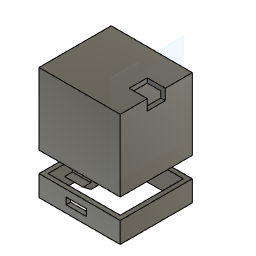
Cover_BoxAndBase (Autodesk Fusion 360 design; units mm, degrees)
Autodesk Fusion 360 part; units mm, degrees
sketch "Sketch1" plane through (0, 0, 0) normal (1, 0, 0) x (0, 1, 0)
  line L0 (0, 0) -> (14.12, 0)
  line L1 (14.12, 0) -> (14.12, 18.38)
  line L2 (14.12, 18.38) -> (0, 18.38)
  line L3 (0, 18.38) -> (0, 0)
  dimension "d1" = 14.12
  dimension "d2" = 18.38
  constraint horizontal L0
  constraint vertical L1
  constraint horizontal L2
  constraint vertical L3
  constraint coincident L0.start L3.end
  measures "d1" distance of L0.start L0.end
  measures "d2" distance of L0.start L2.end
sketch "Sketch2" plane through (6, 0, 0) normal (1, 0, 0) x (0, 1, 0)
  line L0 (0, 18.38) -> (0, 0)
  line L1 (0, 0) -> (14.12, 0)
  line L2 (14.12, 0) -> (14.12, 18.38)
  line L3 (14.12, 18.38) -> (0, 18.38)
  line L4 (2, 2) -> (12.12, 2)
  line L5 (12.12, 2) -> (12.12, 16.38)
  line L6 (12.12, 16.38) -> (2, 16.38)
  line L7 (2, 16.38) -> (2, 2)
  dimension "d5" = -2
sketch "Sketch3" plane through (6, 0, 0) normal (1, 0, 0) x (0, 1, 0)
  line L0 (12.12, 2) -> (2, 2)
  line L1 (2, 2) -> (2, 16.38)
  line L2 (2, 16.38) -> (12.12, 16.38)
  line L3 (12.12, 16.38) -> (12.12, 2)
  line L4 (0, 18.38) -> (0, 0)
  line L5 (0, 0) -> (14.12, 0)
  line L6 (14.12, 0) -> (14.12, 18.38)
  line L7 (14.12, 18.38) -> (0, 18.38)
  line L8 (8.435, 16.4238) -> (5.685, 16.4238)
  line L9 (5.685, 16.4238) -> (5.685, 18.4238)
  line L10 (5.685, 18.4238) -> (8.435, 18.4238)
  line L11 (8.435, 18.4238) -> (8.435, 16.4238)
  line L12 (8.435, 16.4238) -> (5.685, 18.4238) construction
  line L13 (5.685, 16.4238) -> (8.435, 18.4238) construction
  point P0 (7.06, 17.4238)
  dimension "d8" = 2.75
  dimension "d9" = 2
  constraint horizontal L8
  constraint perpendicular L8 L9
  constraint parallel L8 L10
  constraint parallel L9 L11
  constraint coincident L12 P0
  constraint coincident L13 P0
  measures "d8" distance of L9.end L10.end
  measures "d9" distance of L8.end L9.end
sketch "Sketch4" plane through (0, 0, 0) normal (0, -1, 0) x (1, 0, 0)
  line L0 (0, 18.38) -> (0, 0)
  line L1 (0, 0) -> (6, 0)
  line L2 (6, 0) -> (6, 18.38)
  line L3 (6, 18.38) -> (0, 18.38)
  line L4 (1238, -32) -> (1239, -32)
  line L5 (1239, -32) -> (1239, -46.38)
  line L6 (1239, -46.38) -> (1238, -46.38)
  line L7 (1238, -46.38) -> (1238, -32)
  line L8 (-15, 12.38) -> (-16, 12.38)
  line L9 (-16, 12.38) -> (-16, -2)
  line L10 (-16, -2) -> (-15, -2)
  line L11 (-15, -2) -> (-15, 12.38)
  dimension "d14" = 1
  dimension "d15" = 14.38
  dimension "d16" = 1
  dimension "d17" = 14.38
  constraint horizontal L4
  constraint vertical L5
  constraint horizontal L6
  constraint vertical L7
  constraint vertical L9
  constraint perpendicular L8 L9
  constraint horizontal L10
  constraint parallel L9 L11
  measures "d14" distance of L4.start L4.end
  measures "d15" distance of L4.start L6.end
  measures "d16" distance of L8.start L8.end
  measures "d17" distance of L8.start L10.end
sketch "Sketch5" plane through (0, 0, 2) normal (0, 0, 1) x (-1, 0, 0)
  line L0 (-6, -2) -> (-6, -12.12)
  line L1 (-6, -12.12) -> (0, -12.12)
  line L2 (0, -2) -> (-6, -2)
  line L3 (0, -12.12) -> (0, -2)
sketch "Sketch6" plane through (4, 0, 0) normal (1, 0, 0) x (0, 1, 0)
  line L0 (5.685, 18.38) -> (5.685, 16.38)
  line L1 (5.685, 16.38) -> (8.435, 16.38)
  line L2 (8.435, 16.38) -> (8.435, 18.38)
  line L3 (8.435, 18.38) -> (5.685, 18.38)
  line L4 (12.1332, 16.38) -> (12.1332, 1.9861)
  line L5 (12.1336, 16.4249, -4) -> (2.0136, 16.4249, -4)
  line L6 (2.0136, 16.4249, -4) -> (2.0136, 18.4249, -4)
  line L7 (2.0136, 18.4249, -4) -> (12.1336, 18.4249, -4)
  line L8 (12.1336, 18.4249, -4) -> (12.1336, 16.4249, -4)
  dimension "d20" = 10.12
  dimension "d21" = 2
  constraint vertical L4
sketch "Sketch7" plane through (0, 2, 0) normal (0, 1, 0) x (-1, 0, 0)
  line L0 (0, 16.38) -> (-6, 16.38)
  line L1 (-6, 16.38) -> (-6, 2)
  line L2 (-6, 2) -> (0, 2)
  line L3 (0, 2) -> (0, 16.38)
  line L4 (0, 13) -> (-1, 13)
  line L5 (-1, 13) -> (-1, 11)
  line L6 (-1, 11) -> (0, 11)
  line L7 (0, 11) -> (0, 13)
  constraint horizontal L4
  constraint vertical L5
  constraint horizontal L6
  constraint vertical L7
  constraint coincident L3 L4.start
sketch "Sketch8" plane through (0, 2, 0) normal (0, 1, 0) x (-1, 0, 0)
  line L0 (-1, 13) -> (0, 13)
  line L1 (0, 13) -> (0, 16.38)
  line L2 (0, 16.38) -> (-6, 16.38)
  line L3 (-6, 16.38) -> (-6, 2)
  line L4 (-6, 2) -> (0, 2)
  line L5 (0, 2) -> (0, 11)
  line L6 (0, 11) -> (-1, 11)
  line L7 (-1, 11) -> (-1, 13)
  line L8 (-1, 13) -> (-2, 13)
  line L9 (-2, 13) -> (-2, 15.5114)
  line L10 (-2, 15.5114) -> (-1, 15.5114)
  line L11 (-1, 15.5114) -> (-1, 13)
  dimension "d26" = 1
  constraint horizontal L8
  constraint vertical L9
  constraint horizontal L10
  constraint vertical L11
  constraint coincident L0.start L7.end
  measures "d26" distance of L0.start L8.end
sketch "Sketch9" plane through (0, 8.435, 0) normal (0, -1, 0) x (1, 0, 0)
  line L0 (4, 18.38) -> (4, 16.38)
  line L1 (4, 16.38) -> (6, 16.38)
  line L2 (6, 16.38) -> (6, 18.38)
  line L3 (6, 18.38) -> (4, 18.38)
  line L4 (4.1228, 1.37) -> (4.6228, 1.37)
  line L5 (4.6228, 1.37) -> (4.6228, 16.37)
  line L6 (4.6228, 16.37) -> (4.1228, 16.37)
  line L7 (4.1228, 16.37) -> (4.1228, 1.37)
  dimension "d33" = 0.5
  dimension "d34" = 15
  constraint horizontal L4
  constraint vertical L5
  constraint horizontal L6
  constraint vertical L7
  measures "d33" distance of L4.start L4.end
  measures "d34" distance of L4.start L6.end
sketch "Sketch10" plane through (0, 0, 16.38) normal (0, 0, -1) x (1, 0, 0)
  line L0 (2, -2.0136) -> (2, -12.12)
  line L1 (2, -12.12) -> (6, -12.12)
  line L2 (6, -12.12) -> (6, -8.435)
  line L3 (6, -8.435) -> (4, -8.435)
  line L4 (4, -8.435) -> (4, -5.685)
  line L5 (4, -5.685) -> (6, -5.685)
  line L6 (6, -5.685) -> (6, -2)
  line L7 (6, -2) -> (0, -2)
  line L8 (0, -2) -> (0, -2.0136)
  line L9 (0, -2.0136) -> (2, -2.0136)
  line L10 (-1, 5) -> (12, 5)
  line L11 (12, 5) -> (12, 21)
  line L12 (12, 21) -> (-1, 21)
  line L13 (-1, 21) -> (-1, 5)
  dimension "d39" = 13
  constraint horizontal L10
  constraint vertical L11
  constraint horizontal L12
  constraint vertical L13
  measures "d39" distance of L10.start L10.end
extrude "Extrude11" add sketch "Sketch10" along normal blind 20.5 contours L10 L11 L12 L13 makes body 1
sketch "Sketch11" plane through (0, 0, -4.12) normal (0, 0, -1) x (1, 0, 0)
  line L0 (-1, 21) -> (-1, 5)
  line L1 (-1, 5) -> (12, 5)
  line L2 (12, 5) -> (12, 21)
  line L3 (12, 21) -> (-1, 21)
  line L4 (0, 6) -> (11, 6)
  line L5 (11, 6) -> (11, 20)
  line L6 (11, 20) -> (0, 20)
  line L7 (0, 20) -> (0, 6)
  constraint horizontal L4
  constraint vertical L5
  constraint horizontal L6
  constraint vertical L7
extrude "Extrude12" cut sketch "Sketch11" against normal blind 19.5 contours L4 L5 L6 L7 bodies 1
sketch "Sketch12" plane through (0, 0, 0) normal (0, 0, 1) x (1, 0, 0)
  line L0 (12.1825, -11, 14) -> (8, -11, 14)
  line L1 (8, -11, 14) -> (8, -15, 14)
  line L2 (8, -15, 14) -> (12.1825, -15, 14)
  line L3 (12.1825, -15, 14) -> (12.1825, -11, 14)
extrude "Extrude13" cut sketch "Sketch12" along normal blind 5 contours L0 L1 L2 L3 in plane through (0, 0, 14) normal (0, 0, 1) bodies 1
sketch "Sketch13" plane through (0, 0, 16.38) normal (0, 0, 1) x (-1, 0, 0)
  line L0 (-12, 15) -> (-8, 15)
  line L1 (-8, 15) -> (-8, 11)
  line L2 (-8, 11) -> (-12, 11)
  line L3 (-12, 11) -> (-12, 5)
  line L4 (-12, 5) -> (1, 5)
  line L5 (1, 5) -> (1, 21)
  line L6 (1, 21) -> (-12, 21)
  line L7 (-12, 21) -> (-12, 15)
  line L8 (1, 6) -> (-4.6, 6)
  line L9 (-4.6, 6) -> (-4.6, 20)
  line L10 (-4.6, 20) -> (1, 20)
  line L11 (1, 20) -> (1, 6)
  dimension "d46" = 5.6
  dimension "d47" = 14
  constraint horizontal L8
  constraint vertical L9
  constraint horizontal L10
  constraint vertical L11
  measures "d46" distance of L8.start L8.end
  measures "d47" distance of L8.start L10.end
extrude "Extrude14" add sketch "Sketch13" along normal blind 11 contours L5 L8 L9 L10 L11 bodies 1
extrude "Extrude15" cut 1 faces at (2.7333, -15.3333, 27.38) along direction (0, 0, -1) blind 22 on bodies 1 bodies 1
extrude "Extrude16" add 1 faces at (12, -13.6667, 1.92) along direction (1, 0, 0) blind 5 on bodies 1 bodies 1
extrude "Extrude17" cut 1 faces at (11, -12.3333, 1.92) along direction (1, 0, 0) blind 5 on bodies 1 bodies 1
extrude "Extrude18" add 1 faces at (8, -12.3333, 16.0467) along direction (1, 0, 0) blind 5 on bodies 1 bodies 1
extrude "Extrude19" add 1 faces at (4.6, -15.3333, 15.7133) along direction (-1, 0, 0) blind 4 on bodies 1 bodies 1
extrude "Extrude20" add 1 faces at (0.6, -15.3333, 15.7133) along direction (-1, 0, 0) blind 1.6 on bodies 1 bodies 1
extrude "Extrude21" add 1 faces at (-0.3333, -15.3333, 5.38) along direction (0, 0, 1) blind 10 on bodies 1 bodies 1
box "BoxPrimitive1" add length 14 width 1 height 0.5 placed x (0, 1, 0) y (-1, 0, 0) z (0, 0, 1) at (9.5, -20, 0) bodies 1
extrude "Extrude23" add 1 faces at (8.8333, -15.3333, 0.5) along direction (0, 0, 1) blind 15.5 on bodies 1 bodies 1
extrude "Extrude24" cut 1 faces at (8.8333, -15.3333, 0) along direction (0, 0, 1) blind 7.5 on bodies 1 bodies 1
extrude "Extrude25" add 1 faces at (8.8333, -15.3333, 7.5) along direction (0, 0, -1) blind 2.5 on bodies 1 bodies 1
sketch "Sketch15" plane through (0, 0, 0) normal (1, 0, 0) x (0, 1, 0)
sketch "Sketch16" plane through (17, 0, 0) normal (1, 0, 0) x (0, 1, 0)
  line L0 (-15, 14) -> (-15, 16.38)
  line L1 (-15, 16.38) -> (-21, 16.38)
  line L2 (-21, 16.38) -> (-21, -4.12)
  line L3 (-21, -4.12) -> (-5, -4.12)
  line L4 (-5, -4.12) -> (-5, 16.38)
  line L5 (-5, 16.38) -> (-11, 16.38)
  line L6 (-11, 16.38) -> (-11, 14)
  line L7 (-11, 14) -> (-15, 14)
box "BoxPrimitive2" add length 0.5 width 18 height 0.5 placed x (0, 0, 1) y (-1, 0, 0) z (0, -1, 0) at (17, -21, 0) bodies 1
extrude "Extrude26" cut 1 faces at (5, -21.5, 0.1667) along direction (0, 1, 0) blind 16.5 on bodies 1 bodies 1 makes body 2 at (11, -5, 5.7933)
extrude "Extrude27" add 1 faces at (10.6667, -5.3333, -4.12) along direction (0, 0, -1) blind 0.5 on bodies 1 bodies 1
box "BoxPrimitive3" add length 1.5 width 3 height 1 placed x (0, 0, 1) y (-1, 0, 0) z (0, -1, 0) at (8, -21, -3) bodies 1
extrude "Extrude28" cut 1 faces at (6, -22, -2.5) along direction (0, 1, 0) blind 20 on bodies 1 bodies 1
box "BoxPrimitive4" add length 1.5 width 3 height 2 placed x (0, 0, 1) y (-1, 0, 0) z (0, -1, 0) at (7.9158, -6, 0.5) bodies 2
extrude "Extrude29" cut 1 faces at (4.9158, -6.6667, 1.5) along direction (1, 0, 0) blind 0.2 on bodies 2 bodies 2
extrude "Extrude30" cut 1 faces at (7.9158, -6.6667, 1.5) along direction (-1, 0, 0) blind 0.2 on bodies 2 bodies 2
box "BoxPrimitive5" add length 0.2 width 2.6 height 1 placed x (0, -1, 0) y (-1, 0, 0) z (0, 0, -1) at (7.7158, -6, 0.5) bodies 1 2
extrude "Extrude31" cut 1 faces at (5.9824, -6.0667, -0.5) along direction (0, 0, 1) blind 1.2 on bodies 1 bodies 1 makes body 3 at (11, -5, 5.7933)
extrude "Extrude32" add 1 faces at (6.8491, -7.4, 0.5) along direction (0, 0, -1) blind 2.4 on bodies 3 bodies 3
extrude "Extrude33" add 1 faces at (6.8491, -7.4, -1.9) along direction (0, 0, -1) blind 0.5 on bodies 3 bodies 3
box "BoxPrimitive6" add length 1.5 width 3 height 2 placed x (0, 0, 1) y (1, 0, 0) z (0, 1, 0) at (5, -20, 0.5) bodies 3
extrude "Extrude34" cut 1 faces at (8, -19.3333, 1.5) along direction (-1, 0, 0) blind 0.2 on bodies 3 bodies 3
extrude "Extrude35" cut 1 faces at (5, -19.3333, 1.5) along direction (1, 0, 0) blind 0.2 on bodies 3 bodies 3
box "BoxPrimitive7" add length 0.2 width 2.6 height 0.2 placed x (0, 1, 0) y (1, 0, 0) z (0, 0, -1) at (5.2, -20, 0.5) bodies 3
extrude "Extrude36" cut 1 faces at (6.9333, -19.9333, 0.3) along direction (0, 0, 1) blind 0.4 on bodies 3 bodies 3
extrude "Extrude37" add 1 faces at (6.0667, -19.2, 0.5) along direction (0, 0, -1) blind 3.1 on bodies 3 bodies 3
extrude "Extrude38" cut 1 faces at (6.0667, -19.2, -2.6) along direction (0, 0, 1) blind 0.1 on bodies 3 bodies 3
move_body "Move2" bodies 1 to x (1, 0, 0) y (0, 1, 0) z (0, 0, 1) at (0, 0, -3)
move_body "Move3" bodies 3 to x (1, 0, 0) y (0, 1, 0) z (0, 0, 1) at (0, -6, 0)
move_body "Move4" bodies 1 to x (1, 0, 0) y (0, 1, 0) z (0, 0, 1) at (0, -6, 0)
move_body "Move5" bodies 1 to x (1, 0, 0) y (0, 1, 0) z (0, 0, 1) at (8, 0, 0)
move_body "Move6" bodies 3 to x (1, 0, 0) y (0, 1, 0) z (0, 0, 1) at (8, 0, 0)
move_body "Move7" bodies 1 to x (1, 0, 0) y (0, 1, 0) z (0, 0, 1) at (-13, 0, 0)
sketch "Sketch23" plane through (15.8, 0, 0) normal (1, 0, 0) x (0, 1, 0)
  line L0 (-25.8, -2.5) -> (-24, -2.5)
  line L1 (-24, -2.5) -> (-24, 2)
  line L2 (-24, 2) -> (-26, 2)
  line L3 (-26, 2) -> (-26, 0.7)
  line L4 (-26, 0.7) -> (-25.8, 0.7)
  line L5 (-25.8, 0.7) -> (-25.8, -2.5)
  line L6 (-27.8, -1) -> (-25.8, -1)
  line L7 (-25.8, -1) -> (-25.8, -2.5)
  line L8 (-27.8, -1) -> (-25.8, -2.5)
  dimension "d134" = 1.5
  constraint horizontal L6
  constraint vertical L7
  constraint coincident L0.start L5.end
  measures "d134" distance of L0.start L6.end
extrude "Extrude39" add sketch "Sketch23" against normal blind 2.6 contours L5 L6 L7 L8 bodies 3
sketch "Sketch24" plane through (13.1158, 0, 0) normal (-1, 0, 0) x (0, -1, 0)
  line L0 (12.2, 0.7) -> (12.2, -2.4)
  line L1 (12.2, -2.4) -> (14, -2.4)
  line L2 (14, -2.4) -> (14, 2)
  line L3 (14, 2) -> (12, 2)
  line L4 (12, 2) -> (12, 0.7)
  line L5 (12, 0.7) -> (12.2, 0.7)
  line L6 (10.2, -0.9) -> (12.2, -0.9)
  line L7 (12.2, -0.9) -> (12.2, -2.4)
  line L8 (10.2, -0.9) -> (12.2, -2.4)
  dimension "d138" = 1.5
  constraint horizontal L6
  constraint vertical L7
  constraint coincident L0.end L1.start
  measures "d138" distance of L0.end L6.end
extrude "Extrude40" add sketch "Sketch24" against normal blind 2.6 contours L0 L6 L7 L8 bodies 3
extrude "Extrude41" cut 1 faces at (13.9824, -10.8667, -0.9) along direction (0, 0, -1) blind 0.2 on bodies 3 bodies 3
extrude "Extrude42" cut 1 faces at (14.9333, -27.1333, -1) along direction (0, 0, -1) blind 0.2 on bodies 3 bodies 3
move_body "Move8" bodies 1 to x (1, 0, 0) y (0, 1, 0) z (0, 0, 1) at (13, 0, -1)
copy_body "Body->Comp1" bodies 3 removing the originals makes body 4 in component "Component"
extrude "Extrude1" add 1 faces at (17.5, -16.6667, 9.2933) along direction (1, 0, 0) blind 1.5 on bodies 4 bodies 4 in component "Component"
extrude "Extrude2" cut 1 faces at (16.5, -16.6667, 9.2933) along direction (1, 0, 0) blind 1.5 on bodies 4 bodies 4 in component "Component"
extrude "Extrude3" add 1 faces at (15.8, -24.6, 0.0667) along direction (1, 0, 0) blind 1.5 on bodies 4 bodies 4 in component "Component"
extrude "Extrude4" add 1 faces at (15.7158, -13.4, -0.5) along direction (1, 0, 0) blind 1.5 on bodies 4 bodies 4 in component "Component"
extrude "Extrude43" cut 1 faces at (16, -26.6667, -6.5) along direction (1, 0, 0) blind 1.5 on bodies 1 bodies 1
extrude "Extrude44" cut 1 faces at (16, -11.6667, -6.5) along direction (1, 0, 0) blind 1.5 on bodies 1 bodies 1
component "Component" placed x (1, 0, 0) y (0, 1, 0) z (0, 0, 1) at (0, 0, 0)
